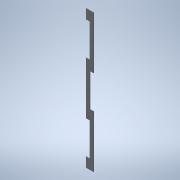
# Autodesk Inventor part: SP56V1 Chapa Detectores
Saved by Autodesk Inventor 2021.2 (Build 252289000, 289)
## iProperties
Created: 2026-10-05
Part Number: SP56V1 Chapa Detectores
Material: Generic
Document SubType Name: Sheet Metal
Designer: nelso
Density: 1 g/cm^3
Sheet Metal Rule: Default_mm
Appearance: Default
Author: nelso
Autodesk Inventor part; units mm, degrees
ref_plane "YZ Plane" through (0, 0, 0) normal (1, 0, 0) x (0, 1, 0)
ref_plane "XZ Plane" through (0, 0, 0) normal (0, 1, 0) x (-1, 0, 0)
ref_plane "XY Plane" through (0, 0, 0) normal (0, 0, 1) x (1, 0, 0)
sketch "Sketch1" plane through (0, 0, 0) normal (0, 1, 0) x (-1, 0, 0)
  line L0 (-30, 565) -> (30, 565) construction
  line L1 (30, 565) -> (30, -565) construction
  line L2 (30, -565) -> (-30, -565) construction
  line L3 (-30, -565) -> (-30, 565) construction
  line L4 (-30, 565) -> (30, -565) construction
  line L5 (30, 565) -> (-30, -565) construction
  line L6 (30, -565) -> (0, -565)
  line L7 (0, -565) -> (0, -485)
  line L8 (0, -485) -> (30, -485)
  line L9 (30, -485) -> (30, -565)
  line L10 (-30, -565) -> (0, -565)
  line L11 (0, -565) -> (0, -135)
  line L12 (0, -135) -> (-30, -135)
  line L13 (-30, -135) -> (-30, -565)
  line L14 (30, -135) -> (30, -215)
  line L15 (30, -215) -> (0, -215)
  line L16 (0, -215) -> (0, 215)
  line L17 (0, 215) -> (30, 215)
  line L18 (30, 215) -> (30, -215)
  line L19 (-30, 565) -> (0, 565)
  line L20 (0, 565) -> (0, 135)
  line L21 (0, 135) -> (-30, 135)
  line L22 (-30, 135) -> (-30, 565)
  line L23 (30, 565) -> (0, 565)
  line L24 (0, 565) -> (0, 485)
  line L25 (0, 485) -> (30, 485)
  line L26 (30, 485) -> (30, 565)
  point P0 (0, 0)
  dimension "d0" = 60
  dimension "d1" = 1130
  dimension "d2" = 80
  dimension "d3" = 430
  dimension "d4" = 80
  dimension "d5" = 430
  dimension "d6" = 430
  dimension "d7" = 80
  measures "d0" distance of L1.end L2.end
  measures "d1" distance of L0.end L1.end
  measures "d2" distance of L6.end L7.end
  measures "d3" distance of L11.end L10.end
  measures "d4" distance of L14.start L14.end
  measures "d5" distance of L15.end L16.end
  measures "d6" distance of L19.end L20.end
  measures "d7" distance of L24.end L23.end
extrude "Plate1" add sketch "Sketch1" along normal blind 3.2
equation "\"d8\" = Thickness"
equation "\"BendReliefWidth\" = Thickness"
equation "\"BendReliefDepth\" = 0.5 * Thickness"
equation "\"CornerReliefSize\" = 4 * Thickness"
equation "\"MinimumRemnant\" = 2 * Thickness"
equation "\"TransitionRadius\" = BendRadius"
equation "\"JacobiRadiusSize\" = BendRadius"
equation "\"GapSize\" = Thickness"
equation "\"Thickness\" = 3.2"
equation "\"BendRadius\" = 1.516"
body "Solid1"
